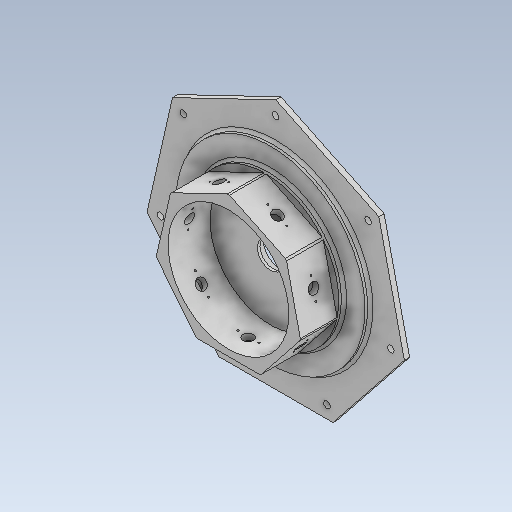
# Autodesk Inventor part: Peça33
Saved by Autodesk Inventor 2021 (Build 250183000, 183)
## iProperties
Category: 41
Created: 2021-07-21
Part Number: Peça33
Material: Genérico
Document SubType Name: Modeling
Designer: Giovanni
Density: 1 g/cm^3
Appearance: Padrão
User Status: 1:8
Author: Giovanni
Keywords: 34
Autodesk Inventor part; units mm, degrees
ref_plane "YZ Plane" through (0, 0, 0) normal (1, 0, 0) x (0, 1, 0)
ref_plane "XZ Plane" through (0, 0, 0) normal (0, 1, 0) x (-1, 0, 0)
ref_plane "XY Plane" through (0, 0, 0) normal (0, 0, 1) x (1, 0, 0)
sketch "Esboço1" plane through (0, 0, 0) normal (0, 0, 1) x (1, 0, 0)
  line L0 (0, 251.2194) -> (196.4112, 156.6327)
  line L1 (196.4112, 156.6327) -> (244.9208, -55.9016)
  line L2 (244.9208, -55.9016) -> (109, -226.3408)
  line L3 (109, -226.3408) -> (-109, -226.3408)
  line L4 (-109, -226.3408) -> (-244.9208, -55.9016)
  line L5 (-244.9208, -55.9016) -> (-196.4112, 156.6327)
  line L6 (-196.4112, 156.6327) -> (0, 251.2194)
  point P0 (0, 0)
  point P1 (0, 0)
  dimension "d0" = 218
  constraints: 14 end point, 1 coincident, 1 horizontal, 15 other
  measures "d0" distance of L2.end L3.end
extrude "Extrusão1" add sketch "Esboço1" along normal blind 10
sketch "Esboço2" plane through (0, 0, 10) normal (0, 0, 1) x (1, 0, 0)
  circle A0 centre (0, 0) radius 180
  dimension "d3" = 360
  constraints: 1 centre point, 1 coincident
  measures "d3" diameter of A0
extrude "Extrusão2" add sketch "Esboço2" along normal blind 10
sketch "Esboço3" plane through (0, 0, 20) normal (0, 0, 1) x (1, 0, 0)
  circle A0 centre (0, 0) radius 180 projected
  circle A1 centre (0, 0) radius 115
  circle A2 centre (0, 0) radius 140
  dimension "d6" = 230
  dimension "d7" = 280
  constraints: 2 centre point, 2 coincident
  measures "d6" diameter of A1
  measures "d7" diameter of A2
extrude "Extrusão3" add sketch "Esboço3" along normal blind 80 contours A2
sketch "Esboço4" plane through (0, 0, 100) normal (0, 0, 1) x (1, 0, 0)
  circle A0 centre (0, 0) radius 140 projected
  circle A1 centre (0, 0) radius 140 projected
  line L0 (-58.9152, -127) -> (58.9152, -127)
  arc A2 (-58.9152, -127) -> (58.9152, -127) centre (0, 0) ccw
  dimension "d10" = 127
  constraints: 4 point on circle, 2 end point, 1 centre point, 1 coincident, 1 concentric, 1 horizontal
  measures "d10" distance from line of L0 A0.centre
extrude "Extrusão4" cut sketch "Esboço4" against normal blind 70 contours L0 A0 picked at (-14.9349, -128.879)
sketch "Esboço5" plane through (-58.9152, -127, 100) normal (0, -1, 0) x (1, 0, 0)
  line L0 (0, 0) -> (117.8304, 0) projected
  circle A0 centre (58.9152, -38) radius 10
  point P0 (58.9152, -100)
  dimension "d13" = 20
  dimension "d14" = 38
  constraints: 1 centre point, 1 vertical alignment
  measures "d13" diameter of A0
  measures "d14" distance from line of A0.centre L0
extrude "Extrusão5" cut sketch "Esboço5" against normal up to surface
sketch "Esboço6" plane through (-58.9152, -127, 100) normal (0, -1, 0) x (1, 0, 0)
  circle A0 centre (58.9152, -38) radius 10 projected
  point P0 (58.9152, -100)
  point P1 (38.9152, -38)
  point P2 (78.9152, -38)
  dimension "d17" = 20
  dimension "d18" = 20
  constraints: 2 horizontal alignment
  measures "d17" distance of A0.centre point (38.915, -38)
  measures "d18" distance of A0.centre point (78.915, -38)
hole "Furo1" at (-20, -127, 62) at (20, -127, 62) direction (0, 1, 0) diameter 3.242 depth 25 tip angle 118 thread size "M4x0.7" class "6H" standard "ANSI Metric M Profile"
pattern_circular "Padrão circular1" count 7 over 360 about axis through (0, 0, 20) along (0, 0, 1) of "Extrusão4", "Extrusão5", "Furo1"
sketch "Esboço7" plane through (0, 0, 0) normal (0, 0, -1) x (-1, 0, 0)
  circle A0 centre (0, 0) radius 34
  dimension "d29" = 68
  constraints: 1 centre point, 1 coincident
  measures "d29" diameter of A0
extrude "Extrusão6" cut sketch "Esboço7" against normal blind 15
sketch "Esboço8" plane through (0, 0, 15) normal (0, 0, -1) x (-1, 0, 0)
  circle A0 centre (0, 0) radius 34 projected
  circle A1 centre (0, 0) radius 25
  dimension "d32" = 50
  constraints: 1 centre point, 1 coincident
  measures "d32" diameter of A1
extrude "Extrusão7" cut sketch "Esboço8" against normal up to next contours A1
sketch "Esboço9" plane through (0, 0, 10) normal (0, 0, 1) x (1, 0, 0)
  circle A0 centre (0, 0) radius 180 projected
  circle A1 centre (0, 225) radius 6.25
  dimension "d35" = 12.5
  dimension "d36" = 225
  constraints: 1 centre point, 1 vertical alignment
  measures "d35" diameter of A1
  measures "d36" distance of A0.centre A1.centre
extrude "Extrusão8" cut sketch "Esboço9" against normal up to next contours A1
pattern_circular "Padrão circular2" count 7 over 360 about axis through (0, 0, -10) along (0, 0, 1) of "Extrusão8"
sketch "Esboço10" plane through (0, 0, 0) normal (0, 0, -1) x (-1, 0, 0)
  circle A0 centre (0, 0) radius 25 projected
  circle A1 centre (0, 0) radius 200
  circle A2 centre (0, 0) radius 190
  dimension "d42" = 400
  dimension "d43" = 380
  constraints: 2 centre point, 1 coincident
  measures "d42" diameter of A1
  measures "d43" diameter of A2
extrude "Extrusão9" add sketch "Esboço10" along normal blind 5 contours A1
fillet "Arredondamento1" radius 5 2 edges at (-180, 0, 10) (-140, 0, 20)
